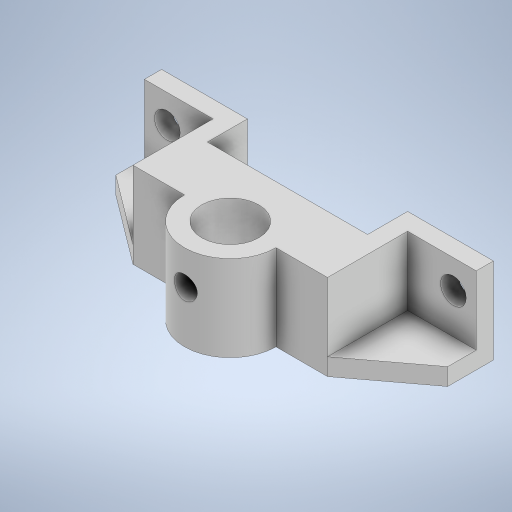
# Autodesk Inventor part: Pen Holder
Saved by Autodesk Inventor 2024 (Build 280153000, 153)
## iProperties
Created: 2023-10-02
Part Number: Pen Holder
Material: Generic
Document SubType Name: Modeling
Designer: ryanm
Density: 1 g/cm^3
Appearance: Default
Author: ryanm
Autodesk Inventor part; units mm, degrees
ref_plane "YZ Plane" through (0, 0, 0) normal (1, 0, 0) x (0, 1, 0)
ref_plane "XZ Plane" through (0, 0, 0) normal (0, 1, 0) x (-1, 0, 0)
ref_plane "XY Plane" through (0, 0, 0) normal (0, 0, 1) x (1, 0, 0)
sketch "Sketch1" plane through (0, 0, 0) normal (0, 1, 0) x (-1, 0, 0)
  line L0 (14, -12.5) -> (29, -12.5)
  line L1 (29, -12.5) -> (29, 12.5)
  line L2 (-29, 12.5) -> (-29, -12.5)
  line L3 (-29, -12.5) -> (-14, -12.5)
  line L4 (-14, -12.5) -> (-14, -5.5)
  line L5 (-14, -5.5) -> (14, -5.5)
  line L6 (14, -5.5) -> (14, -12.5)
  line L7 (29, 12.5) -> (-29, 12.5)
  point P0 (0, 0)
  point P1 (-29, 0)
  point P2 (0, -5.5)
  dimension "d0" = 28
  dimension "d1" = 15
  dimension "d2" = 7
  dimension "d3" = 25
  constraints: 16 end point, 5 perpendicular, 3 vertical alignment, 2 equal length, 2 horizontal, 2 midpoint, 1 horizontal alignment
  measures "d0" distance of L4.end L5.end
  measures "d1" distance of L0.start L0.end
  measures "d2" distance of L5.end L0.start
  measures "d3" distance of L0.end L1.end
extrude "Extrusion1" add sketch "Sketch1" along normal blind 15
sketch "Sketch2" plane through (-29, 0, 12.5) normal (0, 0, 1) x (1, 0, 0)
  line L0 (0, 0) -> (58, 0) projected
  line L1 (58, 0) -> (58, 15) projected
  line L2 (0, 15) -> (58, 15) projected
  line L3 (0, 0) -> (0, 15) projected
  point P0 (29, 0)
  point P1 (4, 10)
  point P2 (54, 10)
  dimension "d6" = 4
  dimension "d7" = 4
  dimension "d8" = 10
  constraints: 1 horizontal alignment
  measures "d6" distance from line of L3 point (4, 10)
  measures "d7" distance from line of L1 point (54, 10)
  measures "d8" distance from line of L0 point (4, 10)
hole "Hole1" at (-25, 10, 12.5) at (25, 10, 12.5) direction (0, 0, -1) diameter 4.5 end through all
sketch "Sketch3" plane through (-29, 0, 12.5) normal (0, 0, 1) x (1, 0, 0)
  circle A0 centre (54, 10) radius 2.25 projected
  circle A1 centre (4, 10) radius 2.25 projected
  line L0 (0, 0) -> (58, 0) projected
  line L1 (58, 0) -> (58, 15) projected
  line L2 (0, 15) -> (58, 15) projected
  line L3 (0, 0) -> (0, 15) projected
  line L4 (12, 15) -> (12, 3)
  line L5 (12, 3) -> (0, 3)
  line L6 (58, 15) -> (43, 15) projected
  line L7 (46, 15) -> (46, 3)
  line L8 (46, 3) -> (58, 3)
  point P0 (29, 0)
  point P1 (15, 15)
  dimension "d16" = 3
  dimension "d17" = 3
  dimension "d18" = 3
  constraints: 8 end point, 4 point on line, 2 perpendicular, 2 vertical, 1 horizontal alignment
  measures "d16" distance from line of point (15, 15) L4
  measures "d17" distance from line of L7 L6.end
  measures "d18" distance between parallel lines of L0 L5
extrude "Extrusion2" cut sketch "Sketch3" against normal blind 22 contours L3 L2 L4 L5 | L8 L7 L2 L1
sketch "Sketch4" plane through (0, 15, 0) normal (0, 1, 0) x (1, 0, 0)
  circle A0 centre (0, -4.5) radius 5
  line L0 (14, 5.5) -> (-14, 5.5) projected
  point P0 (0, 0)
  dimension "d21" = 10
  dimension "d22" = 10
  constraints: 1 centre point, 1 vertical alignment
  measures "d21" diameter of A0
  measures "d22" distance from line of L0 A0.centre
extrude "Extrusion3" cut sketch "Sketch4" against normal through all
sketch "Sketch5" plane through (0, 15, 0) normal (0, 1, 0) x (1, 0, 0)
  circle A0 centre (0, -4.5) radius 5 projected
  circle A1 centre (0, -4.5) radius 8
  line L0 (-8, -4.5) -> (-17, -4.5)
  line L1 (-17, -4.5) -> (-29, 4.5)
  line L2 (-29, 12.5) -> (-29, -12.5) projected
  line L3 (8, -4.5) -> (17, -4.5)
  line L4 (17, -12.5) -> (17, 9.5) projected
  line L5 (17, -4.5) -> (29, 4.5)
  line L6 (29, -12.5) -> (29, 12.5) projected
  line L7 (17, 9.5) -> (29, 9.5) projected
  line L8 (-29, 9.5) -> (-17, 9.5) projected
  line L9 (-17, -12.5) -> (17, -12.5) projected
  line L10 (-17, -12.5) -> (-29, -12.5) projected
  line L11 (-17, -12.5) -> (-17, 9.5) projected
  line L12 (-17, 9.5) -> (-29, 9.5) projected
  line L13 (-29, -12.5) -> (-29, 9.5) projected
  line L14 (29, -12.5) -> (17, -12.5) projected
  line L15 (29, 9.5) -> (29, -12.5) projected
  line L16 (29, 9.5) -> (17, 9.5) projected
  line L17 (17, -12.5) -> (17, 9.5) projected
  point P0 (0, 0)
  point P1 (-29, -12.5)
  point P2 (0, -12.5)
  dimension "d25" = 3
  dimension "d26" = 5
  dimension "d27" = 5
  dimension "d28" = 8
  dimension "d29" = 8
  constraints: 8 end point, 3 point on line, 2 horizontal, 2 point on circle, 1 centre point, 1 vertical alignment
  measures "d25" radial gap between concentric circles of A0 A1
  measures "d26" distance from line of L7 L5.end
  measures "d27" distance from line of L8 L1.end
  measures "d28" distance between parallel lines of L9 L0
  measures "d29" distance between parallel lines of L9 L3
extrude "Extrusion4" cut sketch "Sketch5" against normal through all contours L3 L4 L9 A1 | A1 L9 L11 L0 | L5 L6 L14 L4 | L11 L10 L2 L1
sketch "Sketch6" plane through (0, 0, 0) normal (0, 0, 1) x (1, 0, 0)
  line L0 (17, 3) -> (17, 15) projected
  point P0 (0, 0)
  point P1 (0, 9)
  point P2 (17, 9)
  constraints: 1 horizontal alignment, 1 midpoint, 1 vertical alignment
hole "Hole2" at (0, 9, 0) direction (0, 0, 1) diameter 4 end through all
equation "\"d7\" = d6"
equation "\"d27\" = d26"
equation "\"d29\" = d28"
body "Solid1"
